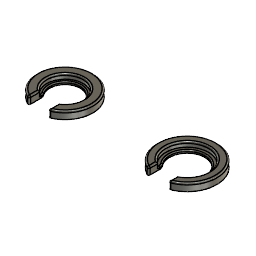
flook32_pipe_clamp (Autodesk Fusion 360 design; units mm, degrees)
Autodesk Fusion 360 part; units mm, degrees
sketch "Sketch1" plane through (0, 0, 0) normal (0, 0, 1) x (1, 0, 0)
  line L0 (-42.0498, -2.7169) -> (-42.0498, -5.115)
  line L1 (-38, -2.7825) -> (-38, -5.1381)
  arc A0 (-37.6659, -1.8041) -> (-42.3664, -1.7615) centre (-40, 0) ccw
  arc A1 (-38, -3.1721) -> (-42.0498, -3.1402) centre (-40, 0) ccw
  arc A2 (-37.5044, -5.4564) -> (-42.5485, -5.4319) centre (-40, 0) ccw
  arc A3 (-42.0498, -2.7169) -> (-42.3664, -1.7615) centre (-43.6498, -2.7169) ccw
  arc A4 (-37.6659, -1.8041) -> (-38, -2.7825) centre (-36.4, -2.7825) ccw
  arc A5 (-42.5485, -5.4319) -> (-42.0498, -5.115) centre (-42.3998, -5.115) ccw
  arc A6 (-38, -5.1381) -> (-37.5044, -5.4564) centre (-37.65, -5.1381) ccw
  line L2 (-57.9546, -3.4271) -> (-57.9546, -6.3405)
  arc A7 (-58.4664, -6.6509) -> (-57.9546, -6.3405) centre (-58.3046, -6.3405) ccw
  line L3 (-52.5, -3.9598) -> (-52.5, -6.5574)
  arc A8 (-52.0509, -2.8483) -> (-58.2761, -2.4651) centre (-55, 0) ccw
  arc A9 (-57.9546, -3.4271) -> (-58.2761, -2.4651) centre (-59.5546, -3.4271) ccw
  arc A10 (-52.5, -6.5574) -> (-52.0105, -6.8784) centre (-52.15, -6.5574) ccw
  arc A11 (-52.0509, -2.8483) -> (-52.5, -3.9598) centre (-50.9, -3.9598) ccw
  arc A12 (-52.0105, -6.8784) -> (-58.4664, -6.6509) centre (-55, 0) ccw
  arc A13 (-52.5, -4.2143) -> (-57.9546, -3.909) centre (-55, 0) ccw
  circle A14 centre (0.4352, 0) radius 5.9
  circle A15 centre (0.4352, 0) radius 7.9
  line L4 (-25.2616, -4.0851) -> (-25.2616, -6.7438)
  arc A16 (-25.2616, -4.0851) -> (-25.6366, -3.0558) centre (-26.8616, -4.0851) ccw
  arc A17 (-18.9331, -3.6272) -> (-25.6366, -3.0558) centre (-22, 0) ccw
  arc A18 (-18.9331, -3.6272) -> (-19.5, -4.849) centre (-17.9, -4.849) ccw
  line L5 (-19.5, -4.849) -> (-19.5, -7.0993)
  arc A19 (-19.5, -7.0993) -> (-19.0196, -7.4241) centre (-19.15, -7.0993) ccw
  arc A20 (-19.0196, -7.4241) -> (-25.7768, -7.0524) centre (-22, 0) ccw
  arc A21 (-25.7768, -7.0524) -> (-25.2616, -6.7438) centre (-25.6116, -6.7438) ccw
  arc A22 (-19.5, -5.1781) -> (-25.2616, -4.7355) centre (-22, 0) ccw
  dimension "d2" = 5.9
  dimension "d3" = 7.5
  dimension "d4" = 12
  dimension "d5" = 1.6
  dimension "d6" = 0.35
  dimension "d28" = 8.2
  dimension "d29" = 9.8
  dimension "d30" = 15
  dimension "d31" = 1.6
  dimension "d32" = 0.35
  dimension "d33" = 11.8
  dimension "d34" = 2
  dimension "d37" = 9.5
  dimension "d38" = 11.5
  dimension "d39" = 16
  dimension "d40" = 1.6
  dimension "d41" = 0.35
  constraint concentric A0 A1
  constraint concentric A0 A2
  constraint vertical L0
  constraint parallel L0 L1
  constraint coincident L0 A1.end
  constraint coincident L1 A1.start
  constraint tangent A0 A3
  constraint tangent L0 A3
  constraint tangent A0 A4
  constraint tangent L1 A4
  constraint equal A3 A4
  constraint tangent L0 A5
  constraint tangent A2 A5
  constraint tangent L1 A6
  constraint tangent A2 A6
  constraint equal A5 A6
  constraint concentric A8 A13
  constraint concentric A8 A12
  constraint vertical L2
  constraint parallel L2 L3
  constraint coincident A13.end L2
  constraint coincident A13.start L3
  constraint tangent A8 A9
  constraint tangent L2 A9
  constraint tangent A8 A11
  constraint tangent L3 A11
  constraint equal A9 A11
  constraint tangent L2 A7
  constraint tangent A7 A12
  constraint tangent L3 A10
  constraint tangent A10 A12
  constraint equal A7 A10
  constraint concentric A17 A22
  constraint concentric A17 A20
  constraint vertical L4
  constraint parallel L4 L5
  constraint coincident A22.end L4
  constraint coincident A22.start L5
  constraint tangent A16 A17
  constraint tangent L4 A16
  constraint tangent A17 A18
  constraint tangent A18 L5
  constraint equal A16 A18
  constraint tangent L4 A21
  constraint tangent A20 A21
  constraint tangent L5 A19
  constraint tangent A19 A20
  constraint equal A19 A21
  measures "d2" diameter of A0
  measures "d3" diameter of A1
  measures "d4" diameter of A2
  measures "d5" radius of A3
  measures "d6" radius of A5
  measures "d28" diameter of A8
  measures "d29" diameter of A13
  measures "d30" diameter of A12
  measures "d31" radius of A9
  measures "d32" radius of A7
  measures "d33" diameter of A14
  measures "d37" diameter of A17
  measures "d38" diameter of A22
  measures "d39" diameter of A20
  measures "d40" radius of A16
  measures "d41" radius of A21
extrude "Extrude1" add sketch "Sketch1" along normal blind 0.7 contours L0 L1 A0 A1 A3 A4 | L2 L3 A8 A9 A11 A13 | L4 A16 A17 A18 L5 A22 makes body 1 at (-38.9736, 3.6068, 0.4667) makes body 2 at (-51.337, -2.8211, 0) makes body 3 at (-18.6252, 4.2232, 0)
extrude "Extrude2" add sketch "Sketch1" along normal blind 2 contours L0 L1 A1 A2 A5 A6 | L2 A7 L3 A10 A12 A13 | L4 L5 A19 A20 A21 A22 bodies 1 2 3
fillet "Fillet1" radius 0.4 18 edges at (-39.9704, 3.7499, 2) (-38, -4.1551, 2) (-37.8391, -5.4326, 2) (-39.9709, 5.9999, 2) (-42.2121, -5.4104, 2) (-42.0498, -4.1276, 2) (-52.5, -5.3858, 2) (-52.3419, -6.8501, 2) (-54.7358, 7.4953, 2) (-58.1231, -6.6398, 2) (-57.9546, -5.1247, 2) (-54.7262, 4.8923, 2) (-21.5596, 5.7331, 2) (-19.5, -6.1387, 2) (-19.346, -7.3892, 2) (-21.5606, 7.9879, 2) (-25.4317, -7.0441, 2) (-25.2616, -5.7396, 2) on bodies 1 2 3
fillet "Fillet2" radius 0.3 15 edges at (-42.131, -2.2136, 0.7) (-39.9733, 2.9499, 0.7) (-37.9142, -2.2656, 0.7) (-38, -2.9773, 0.7) (-42.0498, -2.9285, 0.7) (-57.9546, -3.6681, 0.7) (-58.0371, -2.92, 0.7) (-54.7481, 4.0923, 0.7) (-52.3835, -3.3604, 0.7) (-52.5, -4.087, 0.7) (-25.2616, -4.4103, 0.7) (-25.3582, -3.5373, 0.7) (-21.5966, 4.7328, 0.7) (-19.3514, -4.1755, 0.7) (-19.5, -5.0135, 0.7) on bodies 1 2 3
extrude "Extrude5" add sketch "Sketch1" along normal blind 3 separate body contours A15 makes body 4
hidden bodies 1 4
